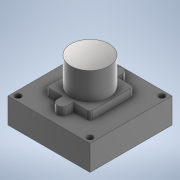
# Autodesk Inventor part: e-CAM50_CUNX
Saved by Autodesk Inventor 2020.4 (Build 244396000, 396)
## iProperties
Part Number: e-CAM50_CUNX
Material: 一般
Document SubType Name: Modeling
Designer: Masato Kubotera
Density: 2.20183 g/cm^3
Appearance: 滑らか - 黒
Mass: 10.8 g
Surface Area: 34.0637 cm^2
Volume: 4.90502 cm^3
Catalog Web Link: https://www.shikino.co.jp/products/product-kbcr-s02mu.php
Description: ReadyMade
Author: Masato Kubotera
Autodesk Inventor part; units mm, degrees
ref_plane "YZ Plane" through (0, 0, 0) normal (1, 0, 0) x (0, 1, 0)
ref_plane "XZ Plane" through (0, 0, 0) normal (0, 1, 0) x (-1, 0, 0)
ref_plane "XY Plane" through (0, 0, 0) normal (0, 0, 1) x (1, 0, 0)
sketch "スケッチ1" plane through (0, 0, 0) normal (0, 0, 1) x (1, 0, 0)
  line L0 (15, 15) -> (-15, 15)
  line L1 (-15, 15) -> (-15, -15)
  line L2 (-15, -15) -> (15, -15)
  line L3 (15, -15) -> (15, 15)
  line L4 (15, 15) -> (-15, -15) construction
  line L5 (-15, 15) -> (15, -15) construction
  line L6 (-13.14, 13.14) -> (13.14, 13.14) construction
  line L7 (13.14, 13.14) -> (13.14, -13.14) construction
  line L8 (13.14, -13.14) -> (-13.14, -13.14) construction
  line L9 (-13.14, -13.14) -> (-13.14, 13.14) construction
  line L10 (-13.14, 13.14) -> (13.14, -13.14) construction
  line L11 (13.14, 13.14) -> (-13.14, -13.14) construction
  circle A0 centre (-13.14, -13.14) radius 1.1
  line L12 (-15, 0) -> (15, 0) construction
  line L13 (0, 15) -> (0, -15) construction
  circle A1 centre (-13.14, 13.14) radius 1.1
  circle A2 centre (13.14, -13.14) radius 1.1
  circle A3 centre (13.14, 13.14) radius 1.1
  circle A4 centre (-13.14, -13.14) radius 2 construction
  circle A5 centre (-13.14, 13.14) radius 2 construction
  circle A6 centre (13.14, -13.14) radius 2 construction
  circle A7 centre (13.14, 13.14) radius 2 construction
  circle A8 centre (0, 0) radius 7
  line L14 (-7, 8) -> (7, 8)
  line L15 (8, 7) -> (8, -7)
  line L16 (7, -8) -> (-7, -8)
  line L17 (-8, -7) -> (-8, 7)
  line L18 (-8, 8) -> (8, -8) construction
  line L19 (8, 8) -> (-8, -8) construction
  arc A9 (-7, 8) -> (-8, 7) centre (-7, 7) ccw
  arc A10 (-8, -7) -> (-7, -8) centre (-7, -7) ccw
  arc A11 (7, -8) -> (8, -7) centre (7, -7) ccw
  arc A12 (8, 7) -> (7, 8) centre (7, 7) ccw
  arc A13 (-10, 2) -> (-10, -2) centre (-10, 0) ccw
  line L20 (-10, 2) -> (-8, 2)
  line L21 (-10, -2) -> (-8, -2)
  arc A14 (10, -2) -> (10, 2) centre (10, 0) ccw
  line L22 (10, 2) -> (8, 2)
  line L23 (10, -2) -> (8, -2)
  point P0 (8, 2)
  point P1 (8, -2)
  dimension "d0" = 30
  dimension "d1" = 30
  dimension "d5" = 2.2
  dimension "d6" = 4
  dimension "d40" = 26.28
  dimension "d41" = 26.28
  dimension "d42" = 14
  dimension "d43" = 16
  dimension "d44" = 16
  dimension "d57" = 1
  dimension "d58" = 2
  dimension "d60" = 20
  constraints: 49 end point, 16 point on line, 15 centre point, 12 midpoint, 12 point on circle, 11 symmetric about line, 9 tangent, 7 parallel, 5 perpendicular, 3 coincident, 3 equal radius, 3 horizontal, 8 other
  measures "d0" distance of L2.end L4.end
  measures "d1" distance of L1.start L4.end
  measures "d5" diameter of A0
  measures "d6" diameter of A4
  measures "d40" distance of L7.end L8.end
  measures "d41" distance of L8.end L6.start
  measures "d42" diameter of A8
  measures "d43" distance of L18.end L19.end
  measures "d44" distance of L19.start L18.end
  measures "d57" radius of A9
  measures "d58" radius of A13
  measures "d60" distance of A14.centre A13.centre
extrude "押し出し1" add sketch "スケッチ1" along normal blind 9.2 contours L3 L2 L1 L0 | A8 | L14 A12 L15 A11 L16 A10 L17 A9 | L17 L21 A13 L20 | L22 A14 L23 L15
extrude "押し出し2" add sketch "スケッチ1" along normal blind 12.2 contours L14 A12 L15 A11 L16 A10 L17 A9 | L17 L21 A13 L20 | L22 A14 L23 L15
extrude "押し出し3" add sketch "スケッチ1" along normal blind 22.2 contours A8
equation "\"d40\" = d41"
equation "\"d44\" = d43"
